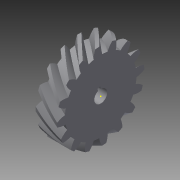
# Autodesk Inventor part: Largegear
Saved by Autodesk Inventor 2015 (Build 190159000, 159)
## iProperties
Created: 2015-09-29
Part Number: Largegear
Material: Generic
Document SubType Name: Modeling
Designer: Ross
Density: 1 g/cm^3
Appearance: Default
Author: Ross
Autodesk Inventor part; units mm, degrees
ref_plane "YZ Plane" through (0, 0, 0) normal (1, 0, 0) x (0, 1, 0)
ref_plane "XZ Plane" through (0, 0, 0) normal (0, 1, 0) x (-1, 0, 0)
ref_plane "XY Plane" through (0, 0, 0) normal (0, 0, 1) x (1, 0, 0)
sketch "Sketch1" plane through (0, 0, 0) normal (1, 0, 0) x (0, 1, 0)
  line L0 (-42.8038, 0) -> (42.8038, 0) projected
  arc A0 (30.5, 1.5) -> (24.8193, 3) centre (23.9043, -11.9721) ccw
  line L1 (30.5, 1.5) -> (30.5, 0)
  arc A1 (24.8193, -3) -> (30.5, -1.5) centre (23.9043, 11.9721) ccw
  line L2 (30.5, -1.5) -> (30.5, 0)
  arc A2 (27.6043, 13.0577) -> (21.782, 12.2696) centre (26.6662, -1.913) ccw
  line L3 (27.6043, 13.0577) -> (28.1783, 11.6718)
  arc A3 (24.0781, 6.7263) -> (28.7524, 10.286) centre (17.5032, 20.2085) ccw
  line L4 (28.7524, 10.286) -> (28.1783, 11.6718)
  arc A4 (20.5061, 22.6274) -> (15.4286, 19.6712) centre (25.3684, 8.4374) ccw
  line L5 (20.5061, 22.6274) -> (21.5668, 21.5668)
  arc A5 (19.6712, 15.4286) -> (22.6274, 20.5061) centre (8.4374, 25.3684) ccw
  line L6 (22.6274, 20.5061) -> (21.5668, 21.5668)
  arc A6 (10.286, 28.7524) -> (6.7263, 24.0781) centre (20.2085, 17.5032) ccw
  line L7 (10.286, 28.7524) -> (11.6718, 28.1783)
  arc A7 (12.2696, 21.782) -> (13.0577, 27.6043) centre (-1.913, 26.6662) ccw
  line L8 (13.0577, 27.6043) -> (11.6718, 28.1783)
  arc A8 (-1.5, 30.5) -> (-3, 24.8193) centre (11.9721, 23.9043) ccw
  line L9 (-1.5, 30.5) -> (0, 30.5)
  arc A9 (3, 24.8193) -> (1.5, 30.5) centre (-11.9721, 23.9043) ccw
  line L10 (1.5, 30.5) -> (0, 30.5)
  arc A10 (-13.0577, 27.6043) -> (-12.2696, 21.782) centre (1.913, 26.6662) ccw
  line L11 (-13.0577, 27.6043) -> (-11.6718, 28.1783)
  arc A11 (-6.7263, 24.0781) -> (-10.286, 28.7524) centre (-20.2085, 17.5032) ccw
  line L12 (-10.286, 28.7524) -> (-11.6718, 28.1783)
  arc A12 (-22.6274, 20.5061) -> (-19.6712, 15.4286) centre (-8.4374, 25.3684) ccw
  line L13 (-22.6274, 20.5061) -> (-21.5668, 21.5668)
  arc A13 (-15.4286, 19.6712) -> (-20.5061, 22.6274) centre (-25.3684, 8.4374) ccw
  line L14 (-20.5061, 22.6274) -> (-21.5668, 21.5668)
  arc A14 (-28.7524, 10.286) -> (-24.0781, 6.7263) centre (-17.5032, 20.2085) ccw
  line L15 (-28.7524, 10.286) -> (-28.1783, 11.6718)
  arc A15 (-21.782, 12.2696) -> (-27.6043, 13.0577) centre (-26.6662, -1.913) ccw
  line L16 (-27.6043, 13.0577) -> (-28.1783, 11.6718)
  arc A16 (-30.5, -1.5) -> (-24.8193, -3) centre (-23.9043, 11.9721) ccw
  line L17 (-30.5, -1.5) -> (-30.5, 0)
  arc A17 (-24.8193, 3) -> (-30.5, 1.5) centre (-23.9043, -11.9721) ccw
  line L18 (-30.5, 1.5) -> (-30.5, 0)
  arc A18 (-27.6043, -13.0577) -> (-21.782, -12.2696) centre (-26.6662, 1.913) ccw
  line L19 (-27.6043, -13.0577) -> (-28.1783, -11.6718)
  arc A19 (-24.0781, -6.7263) -> (-28.7524, -10.286) centre (-17.5032, -20.2085) ccw
  line L20 (-28.7524, -10.286) -> (-28.1783, -11.6718)
  arc A20 (-20.5061, -22.6274) -> (-15.4286, -19.6712) centre (-25.3684, -8.4374) ccw
  line L21 (-20.5061, -22.6274) -> (-21.5668, -21.5668)
  arc A21 (-19.6712, -15.4286) -> (-22.6274, -20.5061) centre (-8.4374, -25.3684) ccw
  line L22 (-22.6274, -20.5061) -> (-21.5668, -21.5668)
  arc A22 (-10.286, -28.7524) -> (-6.7263, -24.0781) centre (-20.2085, -17.5032) ccw
  line L23 (-10.286, -28.7524) -> (-11.6718, -28.1783)
  arc A23 (-12.2696, -21.782) -> (-13.0577, -27.6043) centre (1.913, -26.6662) ccw
  line L24 (-13.0577, -27.6043) -> (-11.6718, -28.1783)
  arc A24 (1.5, -30.5) -> (3, -24.8193) centre (-11.9721, -23.9043) ccw
  line L25 (1.5, -30.5) -> (0, -30.5)
  arc A25 (-3, -24.8193) -> (-1.5, -30.5) centre (11.9721, -23.9043) ccw
  line L26 (-1.5, -30.5) -> (0, -30.5)
  arc A26 (13.0577, -27.6043) -> (12.2696, -21.782) centre (-1.913, -26.6662) ccw
  line L27 (13.0577, -27.6043) -> (11.6718, -28.1783)
  arc A27 (6.7263, -24.0781) -> (10.286, -28.7524) centre (20.2085, -17.5032) ccw
  line L28 (10.286, -28.7524) -> (11.6718, -28.1783)
  arc A28 (22.6274, -20.5061) -> (19.6712, -15.4286) centre (8.4374, -25.3684) ccw
  line L29 (22.6274, -20.5061) -> (21.5668, -21.5668)
  arc A29 (15.4286, -19.6712) -> (20.5061, -22.6274) centre (25.3684, -8.4374) ccw
  line L30 (20.5061, -22.6274) -> (21.5668, -21.5668)
  arc A30 (28.7524, -10.286) -> (24.0781, -6.7263) centre (17.5032, -20.2085) ccw
  line L31 (28.7524, -10.286) -> (28.1783, -11.6718)
  arc A31 (21.782, -12.2696) -> (27.6043, -13.0577) centre (26.6662, 1.913) ccw
  line L32 (27.6043, -13.0577) -> (28.1783, -11.6718)
  arc A32 (24.8193, 3) -> (24.0781, 6.7263) centre (0, 0) ccw
  arc A33 (21.782, 12.2696) -> (19.6712, 15.4286) centre (0, 0) ccw
  arc A34 (15.4286, 19.6712) -> (12.2696, 21.782) centre (0, 0) ccw
  arc A35 (6.7263, 24.0781) -> (3, 24.8193) centre (0, 0) ccw
  arc A36 (-3, 24.8193) -> (-6.7263, 24.0781) centre (0, 0) ccw
  arc A37 (-12.2696, 21.782) -> (-15.4286, 19.6712) centre (0, 0) ccw
  arc A38 (-19.6712, 15.4286) -> (-21.782, 12.2696) centre (0, 0) ccw
  arc A39 (-24.0781, 6.7263) -> (-24.8193, 3) centre (0, 0) ccw
  arc A40 (-24.8193, -3) -> (-24.0781, -6.7263) centre (0, 0) ccw
  arc A41 (-21.782, -12.2696) -> (-19.6712, -15.4286) centre (0, 0) ccw
  arc A42 (-15.4286, -19.6712) -> (-12.2696, -21.782) centre (0, 0) ccw
  arc A43 (-6.7263, -24.0781) -> (-3, -24.8193) centre (0, 0) ccw
  arc A44 (3, -24.8193) -> (6.7263, -24.0781) centre (0, 0) ccw
  arc A45 (12.2696, -21.782) -> (15.4286, -19.6712) centre (0, 0) ccw
  arc A46 (19.6712, -15.4286) -> (21.782, -12.2696) centre (0, 0) ccw
  arc A47 (24.0781, -6.7263) -> (24.8193, -3) centre (0, 0) ccw
  dimension "d1" = 1.5
  dimension "d2" = 15
  dimension "d3" = 3
  dimension "d4" = 30.5
  dimension "d7" = 360
  constraints: 96 point on circle, 64 end point, 48 centre point, 3 symmetric about line, 1 coincident, 1 perpendicular, 1 point on line, 178 other
  measures "d1" distance of L1.start L1.end
  measures "d2" radius of A0
  measures "d3" distance from line of A0.end L0
  measures "d4" distance from line of point (0, 0) L2
coil "Coil1" sketch "Sketch1" operation add axis through (-10, 0, 0) along (1, 0, 0) pitch 200 turns 0.075 hand right
sketch "Sketch2" plane through (15, 26.7341, 0.1851) normal (1, 0, 0) x (0, 0.2115, -0.9774)
  point P0 (-5.4725, -26.1686)
sketch "Sketch3" plane through (15, 26.7341, 0.1851) normal (1, 0, 0) x (0, 0.2115, -0.9774)
  point P0 (-5.4725, -26.1686)
sketch "Sketch4" plane through (15, 26.7341, 0.1851) normal (1, 0, 0) x (0, 0.2115, -0.9774)
  arc A0 (-6.4725, -21.7811) -> (-4.4725, -21.7811) centre (-5.4725, -26.1686) ccw
  line L0 (-5.4725, -26.1686) -> (-5.4725, -21.6686)
  line L1 (-6.4725, -21.6686) -> (-6.4725, -20.6686)
  line L2 (-6.4725, -20.6686) -> (-6.4725, -20.1686)
  line L3 (-6.4725, -20.1686) -> (-4.4725, -20.1686)
  line L4 (-4.4725, -20.1686) -> (-4.4725, -21.7811)
  line L5 (-6.4725, -21.6686) -> (-6.4725, -21.7811)
  dimension "d17" = 9
  dimension "d19" = 1
  dimension "d20" = 1
  dimension "d21" = 0.5
  dimension "d22" = 2
  constraints: 12 end point, 2 perpendicular, 2 point on circle, 1 centre point, 1 coincident, 1 point on line, 1 vertical
  measures "d17" diameter of A0
  measures "d19" distance of L0.end L1.start
  measures "d20" distance of L1.start L1.end
  measures "d21" distance of L1.end L2.end
  measures "d22" distance of L2.end L3.end
extrude "Extrusion1" cut sketch "Sketch4" against normal blind 5
sketch "Sketch5" plane through (10, 26.7341, 0.1851) normal (1, 0, 0) x (0, 0.2115, -0.9774)
  circle A0 centre (-5.4725, -26.1686) radius 4.5
  dimension "d25" = 9
  constraints: 1 centre point, 1 coincident
  measures "d25" diameter of A0
extrude "Extrusion2" cut sketch "Sketch5" against normal blind 15
body "Solid1"
